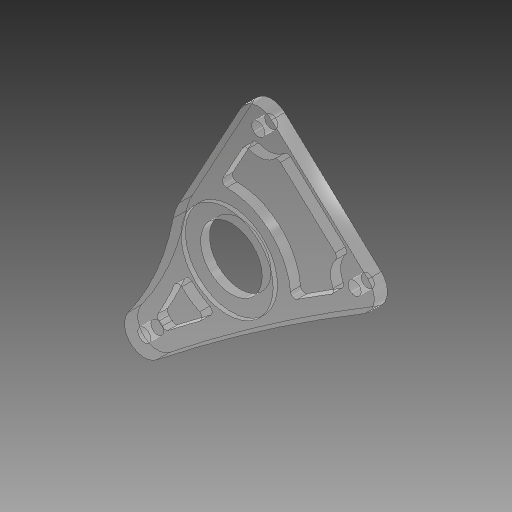
# Autodesk Inventor part: 後脚軸抑え1
Saved by Autodesk Inventor 2020 (Build 240168000, 168)
## iProperties
Created: 2019-09-03
Part Number: 後脚軸抑え1
Material: ポリカーボネート、クリア
Document SubType Name: Modeling
Designer: 雪村
Density: 1.2 g/cm^3
Appearance: ポリカーボネート - クリア
Mass: 3.6709 g
Surface Area: 37.9365 cm^2
Volume: 3.05908 cm^3
Description: ポリカ 3t
Author: 雪村
Autodesk Inventor part; units mm, degrees
ref_plane "YZ Plane" through (0, 0, 0) normal (1, 0, 0) x (0, 1, 0)
ref_plane "XZ Plane" through (0, 0, 0) normal (0, 1, 0) x (-1, 0, 0)
ref_plane "XY Plane" through (0, 0, 0) normal (0, 0, 1) x (1, 0, 0)
sketch "スケッチ1" plane through (0, 0, 0) normal (0, 0, 1) x (1, 0, 0)
  circle A0 centre (119.5841, 99.6659) radius 1.5
  circle A1 centre (141.5641, 79.2483) radius 1.5
  circle A2 centre (112.5, 70) radius 7.025
  circle A3 centre (93.6259, 46.0414) radius 1.5
  circle A4 centre (86.1018, 50.9798) radius 1.5 construction
  circle A5 centre (86.1018, 50.9798) radius 4.5 construction
  circle A6 centre (93.6259, 46.0414) radius 4.5
  circle A7 centre (119.5841, 99.6659) radius 4.5
  circle A8 centre (141.5641, 79.2483) radius 4.5
  circle A9 centre (112.5, 70) radius 12.5
  line L0 (101.529, 75.9907) -> (115.6345, 101.8226)
  line L1 (122.6467, 102.9629) -> (144.6267, 82.5453)
  arc A10 (89.9768, 48.6747) -> (100.2281, 72.3768) centre (41.3227, 83.7856) ccw
  arc A11 (143.8809, 75.3905) -> (96.423, 42.5163) centre (372.805, -305.7819) ccw
  circle A12 centre (112.5, 70) radius 10.5
  point P0 (0, 0)
  point P1 (0, 0)
  dimension "d0" = 9
  dimension "d1" = 9
  dimension "d2" = 9
  dimension "d3" = 9
  dimension "d5" = 60
  dimension "d8" = 3
  dimension "d9" = 3
  dimension "d20" = 21
  dimension "d21" = 2
  constraints: 13 centre point, 12 point on circle, 9 tangent, 5 coincident, 4 end point, 5 other
  measures "d0" diameter of A5
  measures "d1" diameter of A6
  measures "d2" diameter of A7
  measures "d3" diameter of A8
  measures "d5" radius of A10
  measures "d8" diameter of A0
  measures "d9" diameter of A1
  measures "d20" diameter of A12
  measures "d21" radial gap between concentric circles of A12 A9
extrude "押し出し1" add sketch "スケッチ1" along normal blind 3 contours A6 | A6 A10 A9 A11 | A9 | A9 L0 A7 L1 A8 A11 | A8 | A7 | A12
sketch "スケッチ3" plane through (0, 0, 3) normal (0, 0, 1) x (1, 0, 0)
  circle A0 centre (112.5, 70) radius 7.025 projected
  circle A1 centre (112.5, 70) radius 10.5
  point P0 (0, 0)
  dimension "d13" = 21
  constraints: 1 centre point, 1 coincident
  measures "d13" diameter of A1
extrude "押し出し3" cut sketch "スケッチ3" against normal blind 1 contours A0 | A1
shell "シェル1" thickness 4 removed faces 2 at (127.0105, 85.1132, 3) at (126.1434, 84.3451, 0)
fillet "フィレット1" radius 1 14 edges at (96.2217, 50.8903, 1.5) (98.2455, 49.0262, 1.5) (107.8603, 56.2623, 1) (107.8603, 56.2623, 2.5) (126.9919, 69.5148, 2.5) (126.9919, 69.5148, 1) (101.1298, 61.0017, 2.5) (101.1298, 61.0017, 1) (110.6697, 84.384, 1) (110.6697, 84.384, 2.5) (116.5202, 95.0983, 1.5) (123.9373, 96.3045, 1.5) (137.8914, 83.3423, 1.5) (137.1459, 75.9726, 1.5)
sketch "スケッチ4" plane through (0, 0, 0) normal (0, 0, -1) x (-1, 0, 0)
  arc A0 (-128.4875, 70.4902) -> (-136.2992, 75.4486) centre (-372.805, -305.7819) ccw projected
  arc A1 (-136.6631, 76.7522) -> (-136.2992, 75.4486) centre (-135.772, 76.2984) ccw projected
  arc A2 (-136.6631, 76.7522) -> (-137.2584, 82.6704) centre (-141.5641, 79.2483) ccw projected
  arc A3 (-137.1561, 84.0253) -> (-137.2584, 82.6704) centre (-136.4755, 83.2926) ccw projected
  line L0 (-137.1561, 84.0253) -> (-124.6726, 95.6215) projected
  arc A4 (-123.3139, 95.6238) -> (-124.6726, 95.6215) centre (-123.992, 94.8889) ccw projected
  arc A5 (-123.3139, 95.6238) -> (-117.3273, 94.6502) centre (-119.5841, 99.6659) ccw projected
  arc A6 (-116.0393, 94.2175) -> (-117.3273, 94.6502) centre (-116.917, 93.7383) ccw projected
  line L1 (-116.0393, 94.2175) -> (-111.5407, 85.979) projected
  arc A7 (-112.4236, 84.4998) -> (-111.5407, 85.979) centre (-112.4184, 85.4998) ccw projected
  arc A8 (-112.4236, 84.4998) -> (-126.9466, 71.2432) centre (-112.5, 70) ccw projected
  arc A9 (-128.4875, 70.4902) -> (-126.9466, 71.2432) centre (-127.9429, 71.3289) ccw projected
  arc A10 (-100.5355, 59.499) -> (-96.7043, 51.7094) centre (-41.3227, 83.7856) ccw projected
  arc A11 (-96.9629, 50.4133) -> (-96.7043, 51.7094) centre (-97.5696, 51.2082) ccw projected
  arc A12 (-96.9629, 50.4133) -> (-97.6853, 49.7522) centre (-93.6259, 46.0414) ccw projected
  arc A13 (-99.0337, 49.6347) -> (-97.6853, 49.7522) centre (-98.4234, 50.4269) ccw projected
  arc A14 (-99.0337, 49.6347) -> (-106.4215, 55.205) centre (-372.805, -305.7819) ccw projected
  arc A15 (-106.2582, 56.9122) -> (-106.4215, 55.205) centre (-105.8277, 56.0096) ccw projected
  arc A16 (-106.2582, 56.9122) -> (-102.173, 59.8215) centre (-112.5, 70) ccw projected
  arc A17 (-100.5355, 59.499) -> (-102.173, 59.8215) centre (-101.4607, 59.1195) ccw projected
  arc A18 (-96.423, 42.5163) -> (-143.8809, 75.3905) centre (-372.805, -305.7819) ccw projected
  arc A19 (-96.423, 42.5163) -> (-89.9768, 48.6747) centre (-93.6259, 46.0414) ccw projected
  arc A20 (-100.2281, 72.3768) -> (-89.9768, 48.6747) centre (-41.3227, 83.7856) ccw projected
  arc A21 (-100.2281, 72.3768) -> (-101.529, 75.9907) centre (-112.5, 70) ccw projected
  line L2 (-115.6345, 101.8226) -> (-101.529, 75.9907) projected
  arc A22 (-115.6345, 101.8226) -> (-122.6467, 102.9629) centre (-119.5841, 99.6659) ccw projected
  line L3 (-144.6267, 82.5453) -> (-122.6467, 102.9629) projected
  arc A23 (-144.6267, 82.5453) -> (-143.8809, 75.3905) centre (-141.5641, 79.2483) ccw projected
  circle A24 centre (-119.5841, 99.6659) radius 1.5 projected
  circle A25 centre (-141.5641, 79.2483) radius 1.5 projected
  circle A26 centre (-112.5, 70) radius 7.025 projected
  circle A27 centre (-93.6259, 46.0414) radius 1.5 projected
  point P0 (0, 0)
extrude "押し出し4" add sketch "スケッチ4" against normal blind 0.7 contours A0 A1 A2 A3 L0 A4 A5 A6 L1 A7 A8 A9 | A10 A11 A12 A13 A14 A15 A16 A17
sketch "スケッチ5" plane through (0, 0, 3) normal (0, 0, 1) x (1, 0, 0)
  arc A0 (136.2992, 75.4486) -> (128.4875, 70.4902) centre (372.805, -305.7819) ccw projected
  arc A1 (126.9466, 71.2432) -> (128.4875, 70.4902) centre (127.9429, 71.3289) ccw projected
  arc A2 (126.9466, 71.2432) -> (112.4236, 84.4998) centre (112.5, 70) ccw projected
  arc A3 (111.5407, 85.979) -> (112.4236, 84.4998) centre (112.4184, 85.4998) ccw projected
  line L0 (111.5407, 85.979) -> (116.0393, 94.2175) projected
  arc A4 (117.3273, 94.6502) -> (116.0393, 94.2175) centre (116.917, 93.7383) ccw projected
  arc A5 (117.3273, 94.6502) -> (123.3139, 95.6238) centre (119.5841, 99.6659) ccw projected
  arc A6 (124.6726, 95.6215) -> (123.3139, 95.6238) centre (123.992, 94.8889) ccw projected
  line L1 (124.6726, 95.6215) -> (137.1561, 84.0253) projected
  arc A7 (137.2584, 82.6704) -> (137.1561, 84.0253) centre (136.4755, 83.2926) ccw projected
  arc A8 (137.2584, 82.6704) -> (136.6631, 76.7522) centre (141.5641, 79.2483) ccw projected
  arc A9 (136.2992, 75.4486) -> (136.6631, 76.7522) centre (135.772, 76.2984) ccw projected
  arc A10 (106.4215, 55.205) -> (99.0337, 49.6347) centre (372.805, -305.7819) ccw projected
  arc A11 (97.6853, 49.7522) -> (99.0337, 49.6347) centre (98.4234, 50.4269) ccw projected
  arc A12 (97.6853, 49.7522) -> (96.9629, 50.4133) centre (93.6259, 46.0414) ccw projected
  arc A13 (96.7043, 51.7094) -> (96.9629, 50.4133) centre (97.5696, 51.2082) ccw projected
  arc A14 (96.7043, 51.7094) -> (100.5355, 59.499) centre (41.3227, 83.7856) ccw projected
  arc A15 (102.173, 59.8215) -> (100.5355, 59.499) centre (101.4607, 59.1195) ccw projected
  arc A16 (102.173, 59.8215) -> (106.2582, 56.9122) centre (112.5, 70) ccw projected
  arc A17 (106.4215, 55.205) -> (106.2582, 56.9122) centre (105.8277, 56.0096) ccw projected
  circle A18 centre (112.5, 70) radius 10.5 projected
  line L2 (144.6267, 82.5453) -> (122.6467, 102.9629) projected
  arc A19 (122.6467, 102.9629) -> (115.6345, 101.8226) centre (119.5841, 99.6659) ccw projected
  line L3 (115.6345, 101.8226) -> (101.529, 75.9907) projected
  arc A20 (101.529, 75.9907) -> (100.2281, 72.3768) centre (112.5, 70) ccw projected
  arc A21 (89.9768, 48.6747) -> (100.2281, 72.3768) centre (41.3227, 83.7856) ccw projected
  arc A22 (89.9768, 48.6747) -> (96.423, 42.5163) centre (93.6259, 46.0414) ccw projected
  arc A23 (143.8809, 75.3905) -> (96.423, 42.5163) centre (372.805, -305.7819) ccw projected
  arc A24 (143.8809, 75.3905) -> (144.6267, 82.5453) centre (141.5641, 79.2483) ccw projected
  circle A25 centre (119.5841, 99.6659) radius 1.5 projected
  circle A26 centre (141.5641, 79.2483) radius 1.5 projected
  circle A27 centre (93.6259, 46.0414) radius 1.5 projected
  circle A28 centre (112.5, 70) radius 7.025 projected
  point P0 (0, 0)
